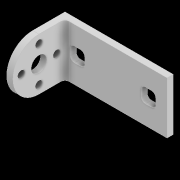
# Autodesk Inventor part: sujetador del motor
Saved by Autodesk Inventor 2020 (Build 240168000, 168)
## iProperties
Created: 2021-11-22
Part Number: sujetador del motor
Material: Generic
Document SubType Name: Modeling
Designer: juan
Density: 1 g/cm^3
Appearance: Default
Author: juan
Autodesk Inventor part; units mm, degrees
ref_plane "YZ Plane" through (0, 0, 0) normal (1, 0, 0) x (0, 1, 0)
ref_plane "XZ Plane" through (0, 0, 0) normal (0, 1, 0) x (-1, 0, 0)
ref_plane "XY Plane" through (0, 0, 0) normal (0, 0, 1) x (1, 0, 0)
sketch "Sketch1" plane through (0, 0, 0) normal (0, 0, 1) x (1, 0, 0)
  line L0 (0, 0) -> (52, 0)
  line L1 (52, 0) -> (52, 25)
  line L2 (52, 25) -> (0, 25)
  line L3 (0, 25) -> (0, 0)
  line L4 (7.4583, 16) -> (10.4583, 16)
  line L5 (12.4583, 14) -> (12.4583, 11)
  line L6 (10.4583, 9) -> (7.4583, 9)
  line L7 (5.4583, 11) -> (5.4583, 14)
  arc A0 (5.4583, 11) -> (7.4583, 9) centre (7.4583, 11) ccw
  arc A1 (7.4583, 16) -> (5.4583, 14) centre (7.4583, 14) ccw
  arc A2 (12.4583, 14) -> (10.4583, 16) centre (10.4583, 14) ccw
  arc A3 (10.4583, 9) -> (12.4583, 11) centre (10.4583, 11) ccw
  line L8 (41.5417, 16) -> (44.5417, 16)
  line L9 (46.5417, 14) -> (46.5417, 11)
  line L10 (44.5417, 9) -> (41.5417, 9)
  line L11 (39.5417, 11) -> (39.5417, 14)
  arc A4 (39.5417, 11) -> (41.5417, 9) centre (41.5417, 11) ccw
  arc A5 (41.5417, 16) -> (39.5417, 14) centre (41.5417, 14) ccw
  arc A6 (46.5417, 14) -> (44.5417, 16) centre (44.5417, 14) ccw
  arc A7 (44.5417, 9) -> (46.5417, 11) centre (44.5417, 11) ccw
  point P0 (12.4583, 9)
  point P1 (12.4583, 16)
  point P2 (5.4583, 9)
  point P3 (5.4583, 12.5)
  point P4 (0, 12.5)
  point P5 (46.5417, 9)
  point P6 (46.5417, 16)
  point P7 (39.5417, 9)
  point P8 (39.5417, 12.5)
  point P9 (12.4583, 12.5)
  dimension "d0" = 52
  dimension "d1" = 25
  dimension "d2" = 7
  dimension "d3" = 7
  dimension "d4" = 2
  dimension "d5" = 5.4583
  dimension "d6" = 7
  dimension "d7" = 7
  dimension "d8" = 2
  dimension "d9" = 5.4583
  constraints: 24 end point, 16 point on circle, 16 tangent, 12 point on line, 8 centre point, 6 equal radius, 6 parallel, 4 midpoint, 3 horizontal, 3 perpendicular, 2 horizontal alignment
  measures "d0" distance of L2.end L1.end
  measures "d1" distance of L0.end L1.end
  measures "d2" distance of point (12.458, 9) point (5.458, 9)
  measures "d3" distance of point (12.458, 16) point (12.458, 9)
  measures "d4" radius of A0
  measures "d5" distance between parallel lines of L3 L7
  measures "d6" distance of point (46.542, 9) point (39.542, 9)
  measures "d7" distance of point (46.542, 16) point (46.542, 9)
  measures "d8" radius of A4
  measures "d9" distance between parallel lines of L1 L9
extrude "Extrusion1" add sketch "Sketch1" along normal blind 3
sketch "Sketch2" plane through (0, 0, 3) normal (0, 0, 1) x (1, 0, 0)
  line L0 (0, 25) -> (0, 0) construction
  line L1 (52, 25) -> (0, 25) construction
  line L2 (0, 0) -> (3, 0)
  line L3 (3, 0) -> (3, 25)
  line L4 (3, 25) -> (0, 25)
  line L5 (0, 25) -> (0, 0)
  dimension "d12" = 3
  constraints: 8 end point, 2 parallel, 1 horizontal, 1 perpendicular, 1 point on line
  measures "d12" distance of L4.end L3.end
extrude "Extrusion2" add sketch "Sketch2" along normal blind 25
sketch "Sketch3" plane through (0, 0, 0) normal (-1, 0, 0) x (0, 0, 1)
  arc A0 (15.5, 0) -> (15.5, 25) centre (15.5, 12.5) ccw
  line L0 (28, 25) -> (28, 0) construction
  line L1 (0, 25) -> (28, 25) construction
  line L2 (15.5, 25) -> (28, 25)
  line L3 (28, 12.5) -> (28, 25)
  line L4 (28, 0) -> (28, 12.5)
  line L5 (15.5, 0) -> (28, 0)
  point P0 (0, 0)
  dimension "d16" = 12.5
  constraints: 8 end point, 4 point on circle, 3 midpoint, 3 tangent, 2 collinear, 2 horizontal alignment, 1 centre point, 1 coincident, 1 horizontal, 1 point on line
  measures "d16" radius of A0
extrude "Extrusion3" cut sketch "Sketch3" against normal blind 25
fillet "Fillet1" radius 2 1 edges at (3, 12.5, 3)
sketch "Sketch4" plane through (0, 0, 0) normal (-1, 0, 0) x (0, 0, 1)
  arc A0 (15.5, 0) -> (15.5, 25) centre (15.5, 12.5) ccw projected
  point P0 (0, 0)
  constraints: 1 coincident
hole "Hole1" at (0, 12.5, 15.5) direction (1, 0, 0) diameter 7.5 end through all
sketch "Sketch5" plane through (0, 0, 0) normal (-1, 0, 0) x (0, 0, 1)
  line L0 (0, 25) -> (0, 0) construction
  circle A0 centre (15.5, 12.5) radius 3.75 construction
  point P0 (15.5, 4)
  dimension "d27" = 15.5
  dimension "d28" = 8.5
  measures "d27" distance from line of L0 point (15.5, 4)
  measures "d28" distance of point (15.5, 4) A0.centre
hole "Hole2" at (0, 4, 15.5) direction (1, 0, 0) diameter 3.4 end through all
pattern_circular "Circular Pattern1" count 4 over 360 about axis through (64.1327, 12.5, 15.5) along (-1, 0, 0) of "Hole2"
equation "\"d9\" = d5"
body "Solid1"
